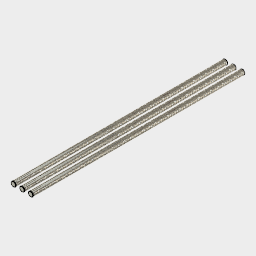
Tower_v7 (Autodesk Fusion 360 archive; units mm, degrees)
design "Z Linear Rods"
Autodesk Fusion 360 part; units mm, degrees
sketch "Sketch1" plane through (0, 0, 0) normal (0, 1, 0) x (1, 0, 0) in component "Z Linear Rod"
  circle A0 centre (0, 0) radius 3
  dimension "d1" = 6
  measures "d1" diameter of A0
extrude "Extrude1" add sketch "Sketch1" along normal mid plane 246 in component "Z Linear Rod"
chamfer "Chamfer1" distance 0.5 angle 45 2 edges at (-2.797, 123, 1.0848) (-2.797, -123, -1.0848) in component "Z Linear Rod"
pattern_linear "R-Pattern1" [suppressed]
component "Z Linear Rod" placed x (1, 0, 0) y (0, 1, 0) z (0, 0, 1) at (0, 0, 0)
component "Z Linear Rod" placed x (1, 0, 0) y (0, 1, 0) z (0, 0, 1) at (10, 0, 0)
component "Z Linear Rod" placed x (1, 0, 0) y (0, 1, 0) z (0, 0, 1) at (20, 0, 0)
